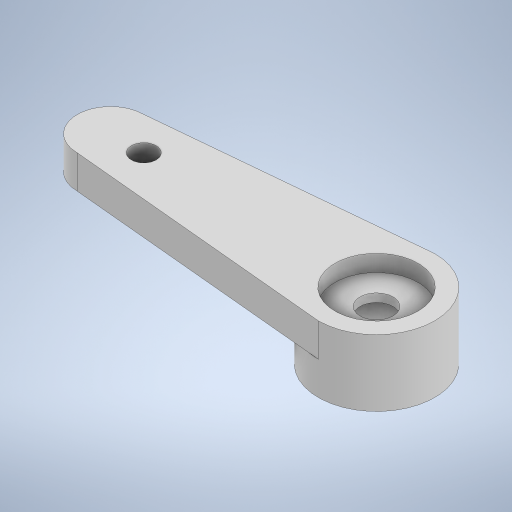
# Autodesk Inventor part: Langbektang houder
Saved by Autodesk Inventor 2023.2 (Build 272271000, 271)
## iProperties
Created: 2020-09-09
Part Number: Langbektang houder
Material: Generic
Document SubType Name: Modeling
Designer: nathan.bollaert
Density: 1 g/cm^3
Appearance: Default
Author: nathan.bollaert
Autodesk Inventor part; units mm, degrees
ref_plane "YZ Plane" through (0, 0, 0) normal (1, 0, 0) x (0, 1, 0)
ref_plane "XZ Plane" through (0, 0, 0) normal (0, 1, 0) x (-1, 0, 0)
ref_plane "XY Plane" through (0, 0, 0) normal (0, 0, 1) x (1, 0, 0)
sketch "Sketch1" plane through (0, 0, 0) normal (0, 1, 0) x (-1, 0, 0)
  circle A0 centre (0, 0) radius 2.5
  circle A1 centre (0, 0) radius 3.5
  dimension "d228" = 5
  dimension "d229" = 7
  constraints: 2 centre point, 2 coincident
  measures "d228" diameter of A0
  measures "d229" diameter of A1
extrude "Extrusion1" add sketch "Sketch1" along normal blind 2
sketch "Sketch2" plane through (0, 2, 0) normal (0, 1, 0) x (1, 0, 0)
  circle A0 centre (0, 0) radius 3.5
  circle A1 centre (0, 0) radius 3.5 projected
  line L0 (-16, -2) -> (0, -3.5)
  circle A2 centre (0, 0) radius 3.5 projected
  line L1 (0, 3.5) -> (-16, 2)
  circle A3 centre (-14, 0) radius 0.75
  arc A4 (-16, 2) -> (-16, -2) centre (-16, 0) ccw
  circle A5 centre (0, 0) radius 1
  circle A6 centre (0, 0) radius 2.5
  circle A7 centre (0, 0) radius 2.5 projected
  dimension "d234" = 1.5
  dimension "d236" = 16
  dimension "d237" = 2
  dimension "d238" = 2
  dimension "d241" = 2
  constraints: 5 centre point, 4 end point, 4 point on circle, 4 vertical alignment, 3 coincident, 2 concentric, 2 horizontal alignment
  measures "d234" diameter of A3
  measures "d236" distance of point (0, 0) A4.centre
  measures "d237" radius of A4
  measures "d238" distance of A4.centre A3.centre
  measures "d241" diameter of A5
extrude "Extrusion2" add sketch "Sketch2" along normal blind 2 contours A0 L0 L1 | A0 L0 A4 L1
extrude "Extrusion3" add sketch "Sketch2" along normal blind 1 contours A6
extrude "Extrusion4" cut sketch "Sketch2" along normal blind 0.5 contours A6
body "Solid5"
